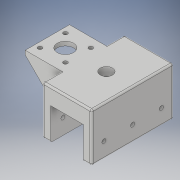
# Autodesk Inventor part: Rahmen_Y_Halterung_v2
Saved by Autodesk Inventor 2019 (Build 230136000, 136)
## iProperties
Created: 2018-08-28
Part Number: Rahmen_Y_Halterung_v2
Material: Generic
Document SubType Name: Modeling
Designer: Julia
Density: 1 g/cm^3
Appearance: Default
Author: Julia
Autodesk Inventor part; units mm, degrees
ref_plane "YZ Plane" through (0, 0, 0) normal (1, 0, 0) x (0, 1, 0)
ref_plane "XZ Plane" through (0, 0, 0) normal (0, 1, 0) x (-1, 0, 0)
ref_plane "XY Plane" through (0, 0, 0) normal (0, 0, 1) x (1, 0, 0)
sketch "Sketch1" plane through (0, 0, 0) normal (0, 1, 0) x (-1, 0, 0)
  line L0 (30, 50) -> (-30, 50)
  line L1 (-30, 50) -> (-30, -50)
  line L2 (-30, -50) -> (30, -50)
  line L3 (30, -50) -> (30, 50)
  point P0 (0, 0)
  point P1 (0, -50)
  point P2 (30, 0)
  dimension "d0" = 100
  dimension "d1" = 60
  constraints: 8 end point, 2 midpoint, 2 parallel, 1 horizontal, 1 horizontal alignment, 1 perpendicular, 1 vertical alignment
  measures "d0" distance of L2.end L0.start
  measures "d1" distance of L1.end L2.end
extrude "Extrusion1" add sketch "Sketch1" along normal blind 20
sketch "Sketch2" plane through (0, 0, 0) normal (0, -1, 0) x (1, 0, 0)
  line L0 (-30, 50) -> (-20, 50)
  line L1 (-20, 50) -> (-20, -50)
  line L2 (-20, -50) -> (-30, -50)
  line L3 (-30, -50) -> (-30, 50)
  line L4 (-30, 50) -> (30, 50) projected
  line L5 (-30, -50) -> (-30, 50) projected
  line L6 (30, -50) -> (-30, -50) projected
  line L7 (20, 50) -> (30, 50)
  line L8 (30, 50) -> (30, -50)
  line L9 (30, -50) -> (20, -50)
  line L10 (20, -50) -> (20, 50)
  line L11 (30, 50) -> (30, -50) projected
  point P0 (0, 0)
  dimension "d4" = 20
  dimension "d6" = 20
  constraints: 16 end point, 6 collinear, 4 parallel, 2 horizontal, 2 perpendicular
  measures "d4" distance from line of L1 point (0, 0)
  measures "d6" distance from line of point (0, 0) L10
extrude "Extrusion2" add sketch "Sketch2" along normal blind 39 contours L0 L1 L2 L3 | L4 L8 L6 L10
sketch "Sketch3" plane through (30, 20, 50) normal (1, 0, 0) x (0, 0, -1)
  line L0 (0, -59) -> (0, 0) projected
  line L1 (100, -59) -> (100, 0) projected
  point P0 (50, -20)
  point P1 (15, -40)
  point P2 (85, -40)
  point P3 (50, -40)
  dimension "d9" = 20
  dimension "d10" = 15
  dimension "d11" = 15
  constraints: 2 horizontal alignment, 1 vertical alignment
  measures "d9" vertical distance of point (50, -20) point (15, -40)
  measures "d10" distance from line of L0 point (15, -40)
  measures "d11" distance from line of L1 point (85, -40)
hole "Hole2" at (30, -20, 35) at (30, -20, -35) at (30, -20, 0) direction (-1, 0, 0) diameter 5 end through all
sketch "Sketch4" plane through (-20, 0, 50) normal (1, 0, 0) x (0, 0, -1)
  line L0 (22.5, -17.5) -> (42.5, -17.5)
  line L1 (42.5, -17.5) -> (42.5, -22.5)
  line L2 (42.5, -22.5) -> (22.5, -22.5)
  line L3 (22.5, -22.5) -> (22.5, -17.5)
  circle A0 centre (50, -20) radius 2.5 projected
  circle A1 centre (15, -20) radius 2.5 projected
  line L4 (57.5, -17.5) -> (77.5, -17.5)
  line L5 (77.5, -17.5) -> (77.5, -22.5)
  line L6 (77.5, -22.5) -> (57.5, -22.5)
  line L7 (57.5, -22.5) -> (57.5, -17.5)
  circle A2 centre (85, -20) radius 2.5 projected
  point P0 (50, 0)
  point P1 (42.5, -20)
  dimension "d26" = 5
  dimension "d27" = 5
  dimension "d28" = 5
  dimension "d29" = 5
  dimension "d30" = 5
  constraints: 16 end point, 4 parallel, 2 collinear, 2 horizontal, 2 perpendicular, 1 horizontal alignment, 1 midpoint
  measures "d26" distance edge to line of A0 L1
  measures "d27" distance edge to line of A1 L3
  measures "d28" distance between parallel lines of L2 L0
  measures "d29" distance edge to line of A0 L7
  measures "d30" distance edge to line of A2 L5
extrude "Extrusion3" add sketch "Sketch4" along normal blind 5 contours L0 L1 L2 L3 | L4 L5 L6 L7
sketch "Sketch5" plane through (20, 0, -50) normal (-1, 0, 0) x (0, 0, 1)
  line L0 (20, -17.5) -> (42.5, -17.5)
  line L1 (42.5, -17.5) -> (42.5, -22.5)
  line L2 (42.5, -22.5) -> (20, -22.5)
  line L3 (20, -22.5) -> (20, -17.5)
  circle A0 centre (15, -20) radius 2.5 projected
  circle A1 centre (50, -20) radius 2.5 projected
  line L4 (57.5, -17.5) -> (77.5, -17.5)
  line L5 (77.5, -17.5) -> (77.5, -22.5)
  line L6 (77.5, -22.5) -> (57.5, -22.5)
  line L7 (57.5, -22.5) -> (57.5, -17.5)
  circle A2 centre (85, -20) radius 2.5 projected
  point P0 (50, 0)
  point P1 (42.5, -20)
  dimension "d33" = 5
  dimension "d34" = 5
  dimension "d35" = 5
  dimension "d36" = 5
  dimension "d37" = 5
  constraints: 16 end point, 4 parallel, 2 collinear, 2 horizontal, 2 perpendicular, 1 horizontal alignment, 1 midpoint
  measures "d33" distance from line of A0.centre L3
  measures "d34" distance edge to line of A1 L1
  measures "d35" distance between parallel lines of L2 L0
  measures "d36" distance edge to line of A1 L7
  measures "d37" distance edge to line of A2 L5
extrude "Extrusion4" add sketch "Sketch5" along normal blind 5 contours L0 L1 L2 L3 | L4 L5 L6 L7
sketch "Sketch6" plane through (-30, 20, -50) normal (-1, 0, 0) x (0, 0, 1)
  line L0 (23, 0) -> (77, 0)
  line L1 (77, 0) -> (77, -5)
  line L2 (77, -5) -> (23, -5)
  line L3 (23, -5) -> (23, 0)
  line L4 (0, 0) -> (100, 0) projected
  point P0 (50, -20)
  point P1 (50, 0)
  dimension "d40" = 5
  dimension "d41" = 54
  constraints: 8 end point, 2 parallel, 1 collinear, 1 horizontal, 1 midpoint, 1 perpendicular, 1 vertical alignment
  measures "d40" distance between parallel lines of L2 L0
  measures "d41" distance between parallel lines of L1 L3
extrude "Extrusion5" add sketch "Sketch6" along normal blind 44
sketch "Sketch7" plane through (-30, -39, -50) normal (-1, 0, 0) x (0, 0, 1)
  line L0 (23, 54) -> (28, 54)
  line L1 (28, 54) -> (28, 10)
  line L2 (28, 10) -> (23, 10)
  line L3 (23, 10) -> (23, 54)
  line L4 (77, 54) -> (23, 54) projected
  line L5 (23, 54) -> (23, 59) projected
  line L6 (72, 54) -> (77, 54)
  line L7 (77, 54) -> (77, 10)
  line L8 (77, 10) -> (72, 10)
  line L9 (72, 10) -> (72, 54)
  line L10 (77, 59) -> (77, 54) projected
  point P0 (50, 39)
  dimension "d44" = 5
  dimension "d45" = 44
  dimension "d46" = 5
  dimension "d47" = 44
  constraints: 16 end point, 4 collinear, 4 parallel, 2 horizontal, 2 perpendicular
  measures "d44" distance between parallel lines of L3 L1
  measures "d45" distance between parallel lines of L0 L2
  measures "d46" distance between parallel lines of L7 L9
  measures "d47" distance between parallel lines of L4 L8
extrude "Extrusion6" add sketch "Sketch7" along normal blind 44
sketch "Sketch10" plane through (-30, 15, -22) normal (0, -1, 0) x (1, 0, 0)
  circle A0 centre (-22, 22) radius 10
  line L0 (-44, 0) -> (-44, 44) projected
  line L1 (0, 44) -> (-44, 44) projected
  point P0 (30, 22)
  point P1 (-37.5, 6.5)
  point P2 (-6.5, 6.5)
  point P3 (-6.5, 37.5)
  point P4 (-37.5, 37.5)
  dimension "d56" = 22
  dimension "d57" = 22
  dimension "d58" = 20
  dimension "d59" = 15.5
  dimension "d60" = 15.5
  dimension "d63" = 360
  constraints: 1 centre point, 5 other
  measures "d56" distance from line of L0 A0.centre
  measures "d57" distance from line of L1 A0.centre
  measures "d58" diameter of A0
  measures "d59" horizontal distance of A0.centre point (-37.5, 6.5)
  measures "d60" horizontal distance of A0.centre point (-37.5, 6.5)
extrude "Extrusion9" cut sketch "Sketch10" against normal up to next
hole "Hole3" at (-67.5, 15, -15.5) at (-36.5, 15, -15.5) at (-36.5, 15, 15.5) at (-67.5, 15, 15.5) direction (0, 1, 0) diameter 5 end through all
chamfer "Chamfer1" distance 44 angle 45 2 edges at (-74, -29, 24.5) (-74, -29, -24.5)
fillet "Fillet1" radius 2 3 edges at (30, 20, 0) (0, 20, 50) (0, 20, -50)
fillet "Fillet2" radius 2 10 edges at (-30, 19.4142, 49.4142) (-30, 20, 37.5) (-30, -10.5, 50) (29.4142, 19.4142, 49.4142) (30, -10.5, 50) (-30, 19.4142, -49.4142) (-30, 20, -37.5) (-30, -10.5, -50) (29.4142, 19.4142, -49.4142) (30, -10.5, -50)
sketch "Sketch12" plane through (0, 0, 0) normal (0, -1, 0) x (1, 0, 0)
  line L0 (-2.5, 27.5) -> (2.5, 27.5)
  line L1 (2.5, 27.5) -> (2.5, 7.5)
  line L2 (2.5, 7.5) -> (-2.5, 7.5)
  line L3 (-2.5, 7.5) -> (-2.5, 27.5)
  line L4 (-20, 27.5) -> (-15, 27.5) projected
  line L5 (-20, 7.5) -> (-15, 7.5) projected
  line L6 (-2.5, -7.5) -> (2.5, -7.5)
  line L7 (2.5, -7.5) -> (2.5, -27.5)
  line L8 (2.5, -27.5) -> (-2.5, -27.5)
  line L9 (-2.5, -27.5) -> (-2.5, -7.5)
  line L10 (-20, -7.5) -> (-15, -7.5) projected
  line L11 (-20, -27.5) -> (-15, -27.5) projected
  point P0 (0, 0)
  point P1 (0, 27.5)
  point P2 (0, -7.5)
  dimension "d79" = 5
  dimension "d80" = 5
  constraints: 16 end point, 4 collinear, 4 parallel, 2 horizontal, 2 midpoint, 2 perpendicular, 2 vertical alignment
  measures "d79" distance of L0.start L0.end
  measures "d80" distance of L7.end L8.end
extrude "Extrusion10" add sketch "Sketch12" along normal blind 5
fillet "Fillet3" radius 2 10 edges at (-29.4142, -39, 49.4142) (-24, -39, 50) (-30, -39, 0) (-29.4142, -39, -49.4142) (-24, -39, -50) (29.4142, -39, 49.4142) (24, -39, 50) (29.4142, -39, -49.4142) (24, -39, -50) (30, -39, 0)
sketch "Sketch13" plane through (0, 20, 0) normal (0, 1, 0) x (1, 0, 0)
  circle A0 centre (-2, 0) radius 7.5
  circle A1 centre (-52, 0) radius 10 projected
  point P0 (0, 0)
  dimension "d84" = 50
  dimension "d85" = 15
  constraints: 1 centre point, 1 horizontal alignment
  measures "d84" distance of A0.centre A1.centre
  measures "d85" diameter of A0
extrude "Extrusion11" cut sketch "Sketch13" against normal blind 10 contours A0
body "Solid1"
